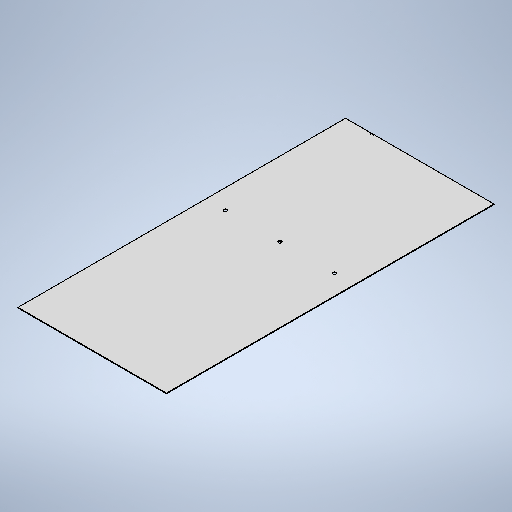
# Autodesk Inventor part: GnG X.6 floor sheet
Saved by Autodesk Inventor 2025.3 (Build 293356030, 356C)
## iProperties
Created: 2025-10-28
Part Number: GnG X.6 floor sheet
Material: Stainless Steel
Document SubType Name: Sheet Metal
Designer: admin
Mass: 24467 g
Surface Area: 20524.5 cm^2
Volume: 3058.37 cm^3
Density: 8 g/cm^3
Sheet Metal Rule: AISI304 3mm Die 32
Sheet Metal Width: 680,000 mm
Sheet Metal Length: 1500,000 mm
Sheet Metal Area: 1020000,000 mm^2
Appearance: Default
Stock Number: O 6
Flat Pattern Width: 68 cm
Flat Pattern Length: 150 cm
Flat Pattern Area: 10200 cm^2
Author: admin
Autodesk Inventor part; units mm, degrees
ref_plane "YZ Plane" through (0, 0, 0) normal (1, 0, 0) x (0, 1, 0)
ref_plane "XZ Plane" through (0, 0, 0) normal (0, 1, 0) x (-1, 0, 0)
ref_plane "XY Plane" through (0, 0, 0) normal (0, 0, 1) x (1, 0, 0)
sketch "Sketch1" plane through (0, 0, 0) normal (0, 0, 1) x (1, 0, 0)
  line L0 (0, 0) -> (-680, 0)
  line L1 (-680, 0) -> (-680, -1500)
  line L2 (-680, -1500) -> (0, -1500)
  line L3 (0, -1500) -> (0, 0)
  line L4 (0, 0) -> (-40, 0)
  line L5 (-40, 0) -> (-40, -35)
  line L6 (-40, -35) -> (0, -35)
  line L7 (0, -35) -> (0, 0)
  line L8 (0, -1500) -> (-40, -1500)
  line L9 (-40, -1500) -> (-40, -1465)
  line L10 (-40, -1465) -> (0, -1465)
  line L11 (0, -1465) -> (0, -1500)
  line L12 (-680, 0) -> (-640, 0)
  line L13 (-640, 0) -> (-640, -35)
  line L14 (-640, -35) -> (-680, -35)
  line L15 (-680, -35) -> (-680, 0)
  line L16 (-680, -1500) -> (-640, -1500)
  line L17 (-640, -1500) -> (-640, -1465)
  line L18 (-640, -1465) -> (-680, -1465)
  line L19 (-680, -1465) -> (-680, -1500)
  line L20 (-240, -1500) -> (-140, -1500)
  line L21 (-140, -1500) -> (-140, -1465)
  line L22 (-140, -1465) -> (-240, -1465)
  line L23 (-240, -1465) -> (-240, -1500)
  line L24 (-240, 0) -> (-140, 0)
  line L25 (-140, 0) -> (-140, -35)
  line L26 (-140, -35) -> (-240, -35)
  line L27 (-240, -35) -> (-240, 0)
  point P0 (0, -35)
  point P1 (-40, 0)
  point P2 (-40, -1500)
  point P3 (0, -1465)
  point P4 (-140, -1500)
  point P5 (-140, 0)
  point P6 (-640, 0)
  point P7 (-680, -35)
  point P8 (-300, -35)
  point P9 (-300, 0)
  point P10 (-260, -2265)
  point P11 (-260, -2300)
  point P12 (-260, -35)
  point P13 (-260, 0)
  point P14 (-300, -2265)
  point P15 (-300, -2300)
  point P16 (-240, 0)
  dimension "d22" = 680
  dimension "d23" = 1500
  dimension "d24" = 40
  dimension "d25" = 35
  dimension "d28" = 100
  dimension "d29" = 100
  measures "d22" distance of L2.end L1.end
  measures "d23" distance of L1.end L0.end
  measures "d24" distance of L6.end L5.end
  measures "d25" distance of L5.end L4.end
  measures "d28" distance of L25.end L26.end
  measures "d29" distance between parallel lines of L5 L25
extrude "Plate1" add sketch "Sketch1" along normal blind 3
sketch "Sketch5" plane through (0, 0, 0) normal (0, 0, -1) x (-1, 0, 0)
  line L0 (680, 0) -> (580, 0) construction
  line L1 (580, 0) -> (580, -2) construction
  line L2 (580, -2) -> (680, -2) construction
  line L3 (680, -2) -> (680, 0) construction
  line L4 (580, 0) -> (578.4752, -4.6556)
  arc A0 (577.5248, -4.6556) -> (578.4752, -4.6556) centre (578, -4.5) ccw
  line L5 (577.5248, -4.6556) -> (576, 0)
  line L6 (576, 0) -> (580, 0)
  line L7 (576, 0) -> (574, 0) construction
  line L8 (574, 0) -> (572, 0)
  line L9 (572, 0) -> (572, -5)
  line L10 (572, -5) -> (574, -5)
  line L11 (574, -5) -> (574, 0)
  line L12 (572, 0) -> (570, 0) construction
  line L13 (570, 0) -> (568, 0)
  line L14 (568, 0) -> (568, -5)
  line L15 (568, -5) -> (570, -5)
  line L16 (570, -5) -> (570, 0)
  line L17 (568, 0) -> (566, 0) construction
  line L18 (566, 0) -> (564, 0)
  line L19 (564, 0) -> (564, -5)
  line L20 (564, -5) -> (566, -5)
  line L21 (566, -5) -> (566, 0)
  line L22 (564, 0) -> (562, 0) construction
  line L23 (562, 0) -> (560, 0)
  line L24 (560, 0) -> (560, -5)
  line L25 (560, -5) -> (562, -5)
  line L26 (562, -5) -> (562, 0)
  line L27 (560, 0) -> (555, 0) construction
  line L28 (555, 0) -> (550, 0) construction
  circle A1 centre (555, 0) radius 1
  circle A2 centre (550, 0) radius 1
  point P0 (0, 0)
  point P1 (578, 0)
  dimension "d30" = 100
  dimension "d31" = 2
  dimension "d32" = 5
  dimension "d33" = 4
  dimension "d34" = 0.5
  dimension "d35" = 5
  dimension "d36" = 5
  dimension "d37" = 5
  dimension "d38" = 2
  constraints: 58 end point, 11 horizontal, 10 equal length, 10 parallel, 5 perpendicular, 4 coincident, 3 centre point, 3 tangent, 2 point on circle, 1 equal radius, 1 midpoint, 1 point on line, 1 vertical alignment
  measures "d30" distance of L2.end L1.end
  measures "d31" distance of L1.end L0.end
  measures "d32" distance of L9.end L9.start
  measures "d33" distance of L5.end L0.end
  measures "d34" radius of A0
  measures "d35" distance of L15.start L13.end
  measures "d36" distance of L19.end L19.start
  measures "d37" distance of L24.end L24.start
  measures "d38" diameter of A1
extrude "Cut1" cut sketch "Sketch5" against normal blind 3 contours L26 L25 L24 L23 | A1 | A2
sketch "Sketch6" plane through (0, 0, 0) normal (0, 0, -1) x (-1, 0, 0)
  circle A0 centre (340, -640) radius 7.5
  arc A1 (549, 0) -> (551, 0) centre (550, 0) ccw projected
  line L0 (554, 0) -> (551, 0) projected
  arc A2 (554, 0) -> (556, 0) centre (555, 0) ccw projected
  line L1 (560, 0) -> (556, 0) projected
  line L2 (560, 0) -> (560, -5) projected
  line L3 (560, -5) -> (562, -5) projected
  line L4 (562, -5) -> (562, 0) projected
  line L5 (680, 0) -> (562, 0) projected
  line L6 (680, -1500) -> (680, 0) projected
  line L7 (0, -1500) -> (680, -1500) projected
  line L8 (0, 0) -> (0, -1500) projected
  line L9 (549, 0) -> (0, 0) projected
  point P0 (340, -1500)
  dimension "d43" = 15
  dimension "d44" = 860
  constraints: 1 centre point, 1 midpoint, 1 vertical alignment
  measures "d43" diameter of A0
  measures "d44" distance from line of A0.centre L7
extrude "Cut2" cut sketch "Sketch6" against normal blind 3 contours A0
pattern_linear "Rectangular Pattern1" count 3 spacing 250 along (1, 0, 0) of "Cut2" first direction both ways yes
equation "\"d33\" = 2 * d31"
equation "\"d34\" = 0.25 * d31"
equation "\"d38\" = d31"
equation "\"d39\" = Thickness"
equation "\"d41\" = Thickness"
equation "\"d2\" = Thickness"
equation "\"BendReliefWidth\" = Thickness"
equation "\"BendReliefDepth\" = 0.5 * Thickness"
equation "\"CornerReliefSize\" = 4 * Thickness"
equation "\"MinimumRemnant\" = 2 * Thickness"
equation "\"TransitionRadius\" = BendRadius"
equation "\"JacobiRadiusSize\" = BendRadius"
equation "\"GapSize\" = Thickness"
equation "\"Thickness\" = 3"
equation "\"BendRadius\" = 5"
body "Solid1"
